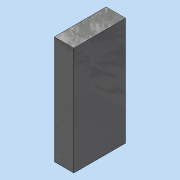
# Autodesk Inventor part: BLANK-BC-10003-A-B
Saved by Autodesk Inventor 2016 (Build 200138000, 138)
## iProperties
Created: 2015-12-02
Part Number: BLANK-BC-10003-A-B
Project: DIPOLO BC-3T- SIRIUS
Cost Center: 1504002005
Material: Aço Carbono
Document SubType Name: Modeling
Designer: reinaldo.basilio
Density: 7.87 g/cm^3
Appearance: Semi-Polished
Mass: 27776 g
Surface Area: 1770.9 cm^2
Volume: 3529.35 cm^3
Description: Polo de baixo campo do dipolo BC-3T lado A-B.
RuleStatus: InUse
AfterMaterialChange0: file://_iMaterial
AfterAnyiPropertyChange0: file://_iMaterial
AfterDocNew0: file://_Naming_par
AfterDocNew1: file://_NameStart
AfterDocNew2: file://_NameStart1
AfterDocNew3: file://_Materiais
DocNumber: XXXXX-XXX-XXXX-00-001.ipt
Folder: .
Title: DIPOLO BC-3T- SIRIUS
Author: reinaldo.basilio
Autodesk Inventor part; units mm, degrees
ref_plane "YZ Plane" through (0, 0, 0) normal (1, 0, 0) x (0, 1, 0)
ref_plane "XZ Plane" through (0, 0, 0) normal (0, 1, 0) x (-1, 0, 0)
ref_plane "XY Plane" through (0, 0, 0) normal (0, 0, 1) x (1, 0, 0)
sketch "Sketch5" plane through (0, 0, 0) normal (0, 0, 1) x (1, 0, 0)
  line L0 (82.5, -31) -> (82.5, 31)
  line L1 (82.5, -31) -> (-82.5, -31)
  line L2 (-82.5, 31) -> (-82.5, -31)
  line L3 (82.5, 31) -> (-82.5, 31)
  circle A0 centre (0, 0) radius 0.4469 construction
  point P0 (0, -31)
  point P1 (82.5, 0)
  dimension "d24" = 62
  dimension "d43" = 165
  constraints: 8 end point, 2 midpoint, 1 centre point, 1 horizontal, 1 horizontal alignment, 1 parallel, 1 perpendicular, 1 vertical alignment, 1 other
  measures "d24" distance between parallel lines of L3 L1
  measures "d43" distance of L0.end L2.start
extrude "Extrusion5" add sketch "Sketch5" along normal mid plane 345
body "Solid5"
